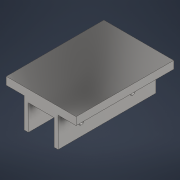
# Autodesk Inventor part: support_basePart_nosleeve
Saved by Autodesk Inventor 2021 (Build 250183000, 183)
## iProperties
Created: 2021-05-24
Part Number: support_basePart_nosleeve
Material: Steel, High Strength, Low Alloy
Document SubType Name: Modeling
Designer: Watchdog
Density: 7.85 g/cm^3
Appearance: Steel - Polished
Author: Watchdog
Autodesk Inventor part; units mm, degrees
ref_plane "YZ Plane" through (0, 0, 0) normal (1, 0, 0) x (0, 1, 0)
ref_plane "XZ Plane" through (0, 0, 0) normal (0, 1, 0) x (-1, 0, 0)
ref_plane "XY Plane" through (0, 0, 0) normal (0, 0, 1) x (1, 0, 0)
sketch "Sketch1" plane through (0, 0, 0) normal (0, 0, 1) x (1, 0, 0)
  line L0 (-33, 0) -> (33, 0)
  line L1 (33, 0) -> (33, -58)
  line L2 (33, -58) -> (-33, -58)
  line L3 (-33, -58) -> (-33, 0)
  point P0 (0, 0)
  dimension "d0" = 58
  dimension "d1" = 66
  dimension "d2" = 33
  dimension "d3" = 0
  constraints: 8 end point, 2 parallel, 1 horizontal, 1 perpendicular
  measures "d0" distance of L2.end L0.start
  measures "d1" distance of L0.start L0.end
  measures "d2" distance from line of point (0, 0) L3
  measures "d3" distance from line of point (0, 0) L0
extrude "clamp_base" add sketch "Sketch1" against normal blind 190
sketch "Sketch2" plane through (0, 0, 0) normal (0, 0, 1) x (1, 0, 0)
  line L0 (-25, -58) -> (25, -58)
  line L1 (25, -58) -> (25, -8)
  line L2 (25, -8) -> (-25, -8)
  line L3 (-25, -8) -> (-25, -58)
  line L4 (-33, -58) -> (33, -58) projected
  point P0 (0, 0)
  dimension "d6" = 50
  dimension "d7" = 50
  dimension "d8" = 25
  constraints: 8 end point, 2 parallel, 1 collinear, 1 horizontal, 1 perpendicular
  measures "d6" distance between parallel lines of L1 L3
  measures "d7" distance of L2.end L0.start
  measures "d8" distance from line of point (0, 0) L3
extrude "clamp_extrusion" cut sketch "Sketch2" against normal through all
sketch "Sketch4" plane through (-33, 0, 0) normal (0, 1, 0) x (1, 0, 0)
  line L0 (-35, 190) -> (101, 190)
  line L1 (101, 190) -> (101, 0)
  line L2 (101, 0) -> (-35, 0)
  line L3 (-35, 0) -> (-35, 190)
  line L4 (66, 0) -> (0, 0) projected
  line L5 (0, 190) -> (66, 190) projected
  line L6 (0, 0) -> (0, 190) projected
  line L7 (66, 0) -> (66, 190) projected
  point P0 (33, 0)
  dimension "d35" = 0
  dimension "d36" = 0
  dimension "d37" = 35
  dimension "d38" = 35
  constraints: 8 end point, 2 parallel, 1 horizontal, 1 perpendicular
  measures "d35" distance between parallel lines of L2 L4
  measures "d36" distance between parallel lines of L0 L5
  measures "d37" distance between parallel lines of L6 L3
  measures "d38" distance between parallel lines of L1 L7
extrude "platform" add sketch "Sketch4" along normal blind 15
sketch "Sketch8" plane through (33, -58, 0) normal (1, 0, 0) x (0, 0, -1)
  line L0 (0, 0) -> (0, 58) projected
  line L1 (190, 58) -> (190, 0) projected
  point P0 (45, 24.0271)
  point P1 (145, 24.0271)
  dimension "d51" = 45
  dimension "d60" = 100
  dimension "d61" = 190
  measures "d51" distance from line of L0 point (45, 24.027)
  measures "d60" distance of point (145, 24.027) point (45, 24.027)
  measures "d61" distance between parallel lines of L1 L0
hole "clampHole" at (33, -33.9729, -45) at (33, -33.9729, -145) direction (-1, 0, 0) diameter 10 end through all
equation "\"d0\" = support_frame_squareBarDimension + support_baseClamp_thickness"
equation "\"d1\" = support_frame_squareBarDimension + 2 * support_baseClamp_thickness"
equation "\"d2\" = 0.5 * d1"
equation "\"d4\" = width"
equation "\"d6\" = support_frame_squareBarDimension"
equation "\"d7\" = support_frame_squareBarDimension"
equation "\"d8\" = 0.5 * d6"
equation "\"d37\" = support_baseClamp_platformLengthBuffer"
equation "\"d38\" = support_baseClamp_platformLengthBuffer"
equation "\"d13\" = support_baseClamp_platformThickness"
equation "\"d51\" = -0.5 * d60 + 0.5 * d61"
equation "\"d60\" = clampHoleSpacing"
equation "\"d53\" = clampHoleDiameter"
equation "\"width\" = clampHoleDiameter + clampHoleSpacing + 2 * buffer"
equation "\"clampHoleSpacing\" = support_frame_clampHoleSpacing"
equation "\"clampHoleDiameter\" = support_frame_clampHoleDiameter"
equation "\"sleeveHoleDiameter\" = support_baseClamp_sleeveHoleDiameter"
equation "\"theta\" = hoop_angle_z"
equation "\"phi\" = support_baseClamp_sleeveSweepTerminationAngle"
equation "\"support_frame_squareBarDimension\" = 50"
equation "\"support_baseClamp_thickness\" = 8"
equation "\"support_baseClamp_sleeveHoleDiameter\" = 12"
equation "\"hoop_angle_z\" = 45deg"
equation "\"support_baseClamp_sleeveSweepTerminationAngle\" = 55deg"
equation "\"support_baseClamp_platformThickness\" = 15"
equation "\"support_baseClamp_platformWidthBuffer\" = 0"
equation "\"support_baseClamp_platformLengthBuffer\" = 35"
equation "\"rack_tooth_thickness\" = 5"
equation "\"rack_tooth_addendum\" = 5"
equation "\"rack_tooth_dedendum\" = 5"
equation "\"hoop_bearing_length\" = 5deg"
equation "\"hoop_cable_diam\" = 5"
equation "\"hoop_cable_pulley_diam\" = 22"
equation "\"secure_arm_radii\" = 9"
equation "\"secure_arm_hold_length\" = 35"
equation "\"secure_arm_angle\" = 20deg"
equation "\"support_frame_endHoleBuffer\" = 25"
equation "\"hoop_tabs_thickness\" = 6"
equation "\"support_frame_squareBarThickness\" = 5"
equation "\"wheelchair_deployed_length\" = 1067"
equation "\"wheelchair_deployed_height\" = 914"
equation "\"hoop_tabs_hole\" = 12"
equation "\"wheelchair_deployed_width\" = 635"
equation "\"support_frame_squareBarFillet\" = 2"
equation "\"sm_varx_pinPlate_thickness\" = 5"
equation "\"sm_varx_member_tolerance\" = 0.5"
equation "\"sm_varx_pinPlate_holeDiameter\" = 5"
equation "\"sm_varx_squareBarThickness\" = 2.5"
equation "\"buffer\" = 40"
equation "\"support_frame_clampHoleSpacing\" = 100"
equation "\"support_frame_clampHoleDiameter\" = 10"
body "Solid1"
